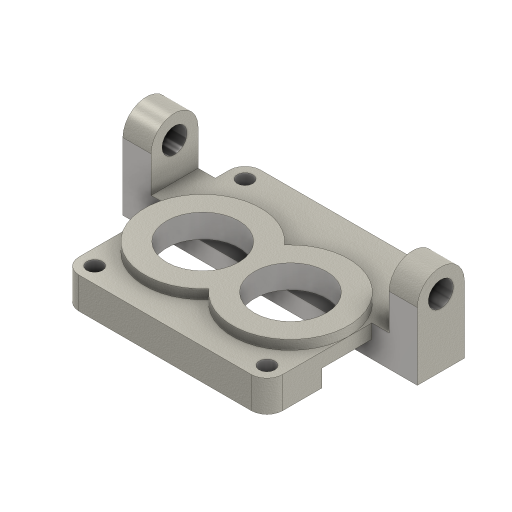
# Autodesk Inventor part: Part023. Cylinder head
Saved by Autodesk Inventor 2023.2 (Build 272271030, 271C)
## iProperties
Created: 2023-09-21
Part Number: Part023. Cylinder head
Material: Steel, Carbon
Document SubType Name: Modeling
Designer: User
Mass: 2442.45 g
Surface Area: 579.069 cm^2
Volume: 311.141 cm^3
Density: 7.85 g/cm^3
Appearance: Steel - Cast
Author: User
Autodesk Inventor part; units mm, degrees
ref_plane "YZ Plane" through (0, 0, 0) normal (1, 0, 0) x (0, 1, 0)
ref_plane "XZ Plane" through (0, 0, 0) normal (0, 1, 0) x (-1, 0, 0)
ref_plane "XY Plane" through (0, 0, 0) normal (0, 0, 1) x (1, 0, 0)
sketch "Sketch1" plane through (0, 0, 0) normal (0, 1, 0) x (-1, 0, 0)
  line L0 (65, -64) -> (-65, -64)
  line L1 (-65, -64) -> (-65, -45)
  line L2 (-65, 52) -> (65, 52)
  line L3 (65, 52) -> (65, -15)
  line L4 (94, -45) -> (65, -45)
  line L5 (65, -45) -> (65, -15) construction
  line L6 (65, -15) -> (94, -15)
  line L7 (94, -15) -> (94, -45)
  line L8 (-65, -45) -> (-94, -45)
  line L9 (-94, -45) -> (-94, -15)
  line L10 (-94, -15) -> (-65, -15)
  line L11 (-65, -15) -> (-65, -30) construction
  line L12 (94, -30) -> (-94, -30) construction
  line L13 (65, -45) -> (65, -64)
  line L14 (65, -15) -> (65, -45) construction
  line L15 (-65, -45) -> (-65, -15) construction
  line L16 (-65, -30) -> (-65, -45) construction
  line L17 (-65, -15) -> (-65, 52)
  point P0 (0, 0)
  point P1 (0, 52)
  dimension "d0" = 116
  dimension "d1" = 130
  dimension "d2" = 52
  dimension "d3" = 30
  dimension "d4" = 30
  dimension "d5" = 188
  constraints: 36 end point, 15 parallel, 5 perpendicular, 3 horizontal, 3 midpoint, 3 point on line, 1 collinear, 1 vertical alignment
  measures "d0" distance of L0.end L2.start
  measures "d1" distance of L0.start L0.end
  measures "d2" distance from line of L2 point (0, 0)
  measures "d3" distance from line of point (0, 0) L12
  measures "d4" distance of L6.end L4.start
  measures "d5" distance between parallel lines of L9 L7
extrude "Extrusion1" add sketch "Sketch1" along normal blind 20
fillet "Fillet1" radius 10 4 edges at (65, 10, 52) (-65, 10, 52) (-65, 10, -64) (65, 10, -64)
sketch "Sketch2" plane through (0, 20, 0) normal (0, 1, 0) x (1, 0, 0)
  line L0 (65, 15) -> (94, 15) projected
  line L1 (94, 15) -> (94, 45) projected
  line L2 (94, 45) -> (65, 45) projected
  line L3 (94, 15) -> (94, 45) projected
  line L4 (65, 15) -> (94, 15) projected
  line L5 (94, 45) -> (76, 45)
  line L6 (76, 45) -> (76, 15)
  line L7 (76, 15) -> (94, 15)
  line L8 (94, 15) -> (94, 45)
  point P0 (0, 0)
  dimension "d9" = 18
  constraints: 8 end point, 2 parallel, 1 horizontal, 1 perpendicular, 1 point on line
  measures "d9" distance of L7.end L6.end
extrude "Extrusion2" add sketch "Sketch2" along normal blind 38
fillet "Fillet2" radius 15 2 edges at (85, 58, -15) (85, 58, -45)
mirror "Mirror1" about plane through (0, 0, 0) normal (1, 0, 0) of "Extrusion2", "Fillet2"
sketch "Sketch3" plane through (94, 0, -15) normal (1, 0, 0) x (0, 0, -1)
  arc A0 (30, 43) -> (0, 43) centre (15, 43) ccw projected
  point P0 (-15, 0)
  constraints: 1 coincident
hole "Hole1" at (94, 43, -30) direction (-1, 0, 0) diameter 16 end through all
sketch "Sketch4" plane through (0, 20, 0) normal (0, 1, 0) x (1, 0, 0)
  line L0 (-55, -52) -> (55, -52) projected
  arc A0 (0, 24.1868) -> (0, -24.1868) centre (-28, 0) ccw
  line L1 (55, 64) -> (-55, 64) projected
  line L2 (0, 64) -> (0, -52) construction
  arc A1 (0, -24.1868) -> (0, 24.1868) centre (28, 0) ccw
  point P0 (0, 0)
  dimension "d20" = 74
  dimension "d21" = 56
  constraints: 4 point on circle, 2 centre point, 2 end point, 2 midpoint, 2 point on line, 1 horizontal alignment, 1 symmetric about line, 1 other
  measures "d20" diameter of A0
  measures "d21" distance of A1.centre A0.centre
extrude "Extrusion3" add sketch "Sketch4" along normal blind 6
sketch "Sketch5" plane through (0, 26, 0) normal (0, 1, 0) x (1, 0, 0)
  arc A0 (0, 24.1868) -> (0, -24.1868) centre (-28, 0) ccw projected
  point P0 (0, 0)
  constraints: 1 coincident
hole "Hole2" at (-28, 26, 0) direction (0, -1, 0) diameter 46 depth 15
sketch "Sketch6" plane through (0, 26, 0) normal (0, 1, 0) x (1, 0, 0)
  arc A0 (0, -24.1868) -> (0, 24.1868) centre (28, 0) ccw projected
  point P0 (0, 0)
  point P1 (28, 0)
  constraints: 1 coincident
hole "Hole3" at (28, 26, 0) direction (0, -1, 0) diameter 46 depth 15
sketch "Sketch7" plane through (65, 0, -15) normal (1, 0, 0) x (0, 0, -1)
  line L0 (-57, 0) -> (0, 0) projected
  line L1 (0, 0) -> (0, 20) projected
  line L2 (0, 0) -> (-32, 0)
  line L3 (-32, 0) -> (-32, 11)
  line L4 (-32, 11) -> (0, 11)
  line L5 (0, 11) -> (0, 0)
  point P0 (-15, 0)
  point P1 (0, 11)
  dimension "d38" = 32
  dimension "d39" = 11
  constraints: 8 end point, 2 parallel, 1 horizontal, 1 perpendicular
  measures "d38" distance between parallel lines of L1 L3
  measures "d39" distance between parallel lines of L0 L4
extrude "Extrusion4" cut sketch "Sketch7" against normal through all
sketch "Sketch8" plane through (0, 20, 0) normal (0, 1, 0) x (1, 0, 0)
  arc A0 (65, 54) -> (55, 64) centre (55, 54) ccw projected
  arc A1 (-55, 64) -> (-65, 54) centre (-55, 54) ccw projected
  arc A2 (-65, 0) -> (0, -24.1868) centre (-28, 0) ccw projected
  line L0 (-65, 0) -> (-65, -42) projected
  arc A3 (-65, -42) -> (-55, -52) centre (-55, -42) ccw projected
  line L1 (-55, -52) -> (55, -52) projected
  arc A4 (55, -52) -> (65, -42) centre (55, -42) ccw projected
  line L2 (65, -42) -> (65, 0) projected
  arc A5 (0, -24.1868) -> (65, 0) centre (28, 0) ccw projected
  point P0 (0, 0)
hole "Hole4" at (-55, 20, -54) at (55, 20, -54) at (55, 20, 42) at (-55, 20, 42) direction (0, -1, 0) diameter 10 end through all
body "Solid1"
